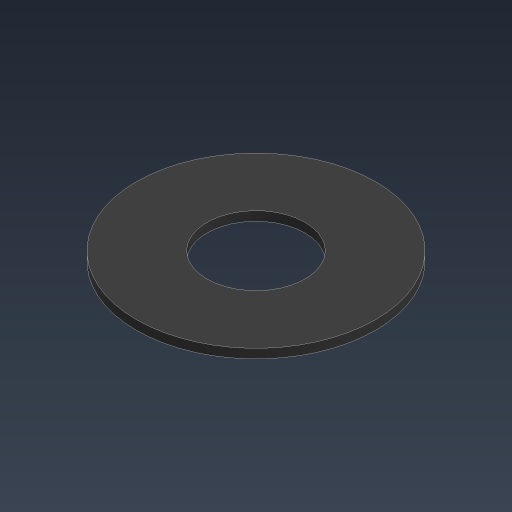
# Autodesk Inventor part: tomites
Saved by Autodesk Inventor 2024.3 (Build 283343000, 343)
## iProperties
Created: 2025-10-06
Part Number: tomites
Material: Rubber
Document SubType Name: Modeling
Designer: Agi
Density: 0.93 g/cm^3
Appearance: Rubber - Black
Author: Agi
Autodesk Inventor part; units mm, degrees
ref_plane "YZ Plane" through (0, 0, 0) normal (1, 0, 0) x (0, 1, 0)
ref_plane "XZ Plane" through (0, 0, 0) normal (0, 1, 0) x (-1, 0, 0)
ref_plane "XY Plane" through (0, 0, 0) normal (0, 0, 1) x (1, 0, 0)
sketch "Sketch1" plane through (0, 0, 0) normal (1, 0, 0) x (0, 1, 0)
  line L0 (0, 16) -> (3, 16)
  line L1 (3, 16) -> (3, 39)
  line L2 (3, 39) -> (0, 39)
  line L3 (0, 39) -> (0, 16)
  line L4 (-0.6, 0) -> (3.6, 0) projected
  point P0 (0, 0)
  point P1 (0, 0)
  dimension "d2" = 3
  dimension "d3" = 23
  constraints: 8 end point, 2 parallel, 1 coincident, 1 horizontal, 1 perpendicular, 1 other
  measures "d2" distance of L2.end L1.end
  measures "d3" distance of L2.end L0.start
revolve "Revolution1" add sketch "Sketch1" angle 360 about axis through (0, -10, 0) along (0, 1, 0)
body "Solid1"
